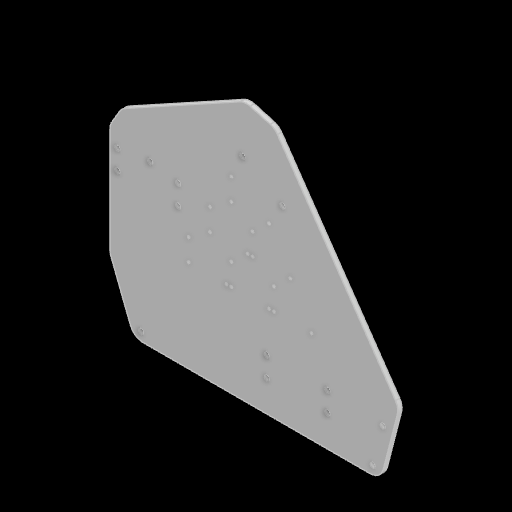
# Autodesk Inventor part: SideChestPanel
Saved by Autodesk Inventor 2025.2 (Build 292293000, 293)
## iProperties
Created: 2025-10-06
Part Number: SideChestPanel
Material: Generic
Document SubType Name: Sheet Metal
Designer: valer
Density: 1 g/cm^3
Sheet Metal Rule: Default
Appearance: Default
Author: valer
Autodesk Inventor part; units mm, degrees
ref_plane "YZ Plane" through (0, 0, 0) normal (1, 0, 0) x (0, 1, 0)
ref_plane "XZ Plane" through (0, 0, 0) normal (0, 1, 0) x (-1, 0, 0)
ref_plane "XY Plane" through (0, 0, 0) normal (0, 0, 1) x (1, 0, 0)
sketch "Base" plane through (0, 0, 0) normal (0, 0, 1) x (1, 0, 0)
  line L0 (-369.2095, 78.4317) -> (-369.2095, 230.2169)
  line L1 (-369.2095, 230.2169) -> (-204.7658, 320.7677)
  line L2 (-204.7658, 320.7677) -> (-168.3839, 310.4358)
  line L3 (-168.3839, 310.4358) -> (-16.9913, 90.7675)
  line L4 (-16.9913, 90.7675) -> (-39.3108, 4.1742)
  line L5 (-39.3108, 4.1742) -> (-340.1274, 4.1742)
  line L6 (-340.1274, 4.1742) -> (-369.2095, 78.4317)
  line L7 (-192.6451, 258.828) -> (-388.2049, 151.1432) construction
  line L8 (-369.2095, 206.6975) -> (-369.2095, 78.4317)
  line L9 (-389.1847, 101.2829) -> (-389.1847, 49.3817) construction
  point P0 (0, 0)
extrude "Plate1" add sketch "Base" along normal blind 5
chamfer "OutsideChamfersFeature" distance 16 angle 45 1 edges at (-369.2095, 230.2169, 2.5)
sketch "MountHoles" plane through (0, 0, 0) normal (0, 0, -1) x (-1, 0, 0)
  line L0 (8.9217, 5.8482) -> (372.782, 5.8482) construction
  line L1 (373.0732, 23.2472) -> (11.408, 23.2472) construction
  line L2 (201.834, 275.5154) -> (397.3937, 167.8305) construction
  line L3 (192.6451, 258.828) -> (388.2049, 151.1432) construction
  line L4 (189.9279, 260.2103) -> (12.2354, 11.4408) construction
  line L5 (169.8355, 264.8558) -> (11.397, 43.0419) construction
  line L6 (290.425, 204.9856) -> (299.6138, 221.673) construction
  line L7 (192.2406, 23.2472) -> (192.2406, 5.8482) construction
  line L8 (101.0816, 135.8256) -> (85.58, 146.8981) construction
  line L9 (340.1274, 4.1742) -> (369.2095, 78.4317) construction
  line L10 (344.19, 14.5477) -> (36.6371, 14.5477) construction
  line L11 (39.3108, 4.1742) -> (16.9913, 90.7675) construction
  line L12 (392.7993, 159.4869) -> (197.2395, 267.1717) construction
  line L13 (388.2049, 151.1432) -> (397.3937, 167.8305) construction
  line L14 (159.0105, 233.3134) -> (27.6512, 49.4103) construction
  circle A0 centre (331.3026, 14.5477) radius 3
  circle A1 centre (49.0293, 14.5477) radius 3
  circle A2 centre (320.285, 199.4168) radius 3
  circle A3 centre (207.7512, 261.3835) radius 3
  circle A4 centre (36.7574, 62.159) radius 3
  circle A5 centre (159.0105, 233.3134) radius 3
  line L15 (355.1938, 237.9346) -> (204.7658, 320.7677) projected
  line L16 (355.1938, 237.9346) -> (326.2023, 185.2849) construction
  point P0 (0, 0)
  point P1 (192.2406, 14.5477)
  point P2 (295.0194, 213.3293)
  point P3 (93.3308, 141.3618)
  dimension "d9" = 6
  dimension "d10" = 12
  dimension "d11" = 12
  dimension "d12" = 12
  dimension "d13" = 12
  dimension "d14" = 12
  constraints: 28 end point, 12 point on line, 10 midpoint, 6 centre point, 5 equal radius, 4 perpendicular, 3 horizontal, 1 coincident, 1 parallel, 16 other
  measures "d9" diameter of A0
  measures "d10" distance from line of A0.centre L9
  measures "d11" distance from line of A1.centre L11
  measures "d12" distance from line of A4.centre L11
  measures "d13" distance of L12.end A3.centre
  measures "d14" distance from line of L16 A2.centre
extrude "MountHolesFeature" cut sketch "MountHoles" against normal blind 5
fillet "OutsideFilletsFeature" radius 16 8 edges at (-340.1274, 4.1742, 2.5) (-369.2095, 78.4317, 2.5) (-39.3108, 4.1742, 2.5) (-16.9913, 90.7675, 2.5) (-168.3839, 310.4358, 2.5) (-204.7658, 320.7677, 2.5) (-355.1938, 237.9346, 2.5) (-369.2095, 214.2169, 2.5)
sketch "HardwareMountHoles" plane through (0, 0, 0) normal (0, 0, -1) x (-1, 0, 0)
  circle A0 centre (175.3952, 206.6354) radius 1.5 projected
  circle A1 centre (221.3566, 233.1714) radius 1.5 projected
  circle A2 centre (149.4146, 161.6352) radius 1.5 projected
  circle A3 centre (195.3761, 161.6353) radius 1.5 projected
  circle A4 centre (195.3761, 188.1712) radius 1.5 projected
  circle A5 centre (221.3567, 206.6355) radius 1.5 projected
  circle A6 centre (201.3761, 161.6355) radius 1.5
  circle A7 centre (247.3376, 161.6357) radius 1.5
  circle A8 centre (247.3375, 188.1716) radius 1.5
  circle A9 centre (227.3571, 116.6357) radius 1.5
  circle A10 centre (273.3186, 116.6361) radius 1.5
  circle A11 centre (273.3184, 143.172) radius 1.5
  circle A12 centre (175.3956, 116.6353) radius 1.5
  circle A13 centre (221.3571, 116.6356) radius 1.5
  circle A14 centre (221.3569, 143.1715) radius 1.5
  circle A15 centre (123.4341, 116.635) radius 1.5
  circle A16 centre (169.3956, 116.6352) radius 1.5
  circle A17 centre (169.3954, 143.1711) radius 1.5
  circle A18 centre (178.2095, 66.1742) radius 3
  circle A19 centre (104.2095, 66.1742) radius 3
  circle A20 centre (104.2095, 42.1742) radius 3
  circle A21 centre (178.2095, 42.1742) radius 3
  circle A22 centre (286.2095, 193.749) radius 3
  circle A23 centre (286.2095, 169.749) radius 3
  circle A24 centre (360.2095, 193.749) radius 3
  circle A25 centre (360.2095, 169.749) radius 3
  point P0 (0, 0)
  constraints: 20 centre point, 40 other
extrude "HardwareMountHolesFeature" cut sketch "HardwareMountHoles" against normal blind 5
equation "\"d15\" = Thickness"
equation "\"d24\" = Thickness"
equation "\"d0\" = Thickness"
equation "\"BendRadius\" = Thickness"
equation "\"BendReliefWidth\" = Thickness"
equation "\"BendReliefDepth\" = 0.5 * Thickness"
equation "\"TransitionRadius\" = BendRadius"
equation "\"JacobiRadiusSize\" = BendRadius"
equation "\"GapSize\" = Thickness"
equation "\"Thickness\" = 5"
body "Solid1"
